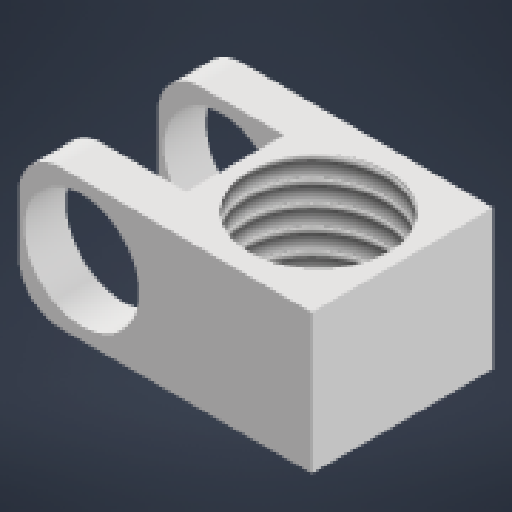
# Autodesk Inventor part: konik
Saved by Autodesk Inventor 2027 (Build 310192060, 192F)
## iProperties
Created: 2026-05-26
Part Number: konik
Material: Ogólny
Document SubType Name: Modeling
Designer: User
Density: 1 g/cm^3
Appearance: Domyślna
Author: User
Autodesk Inventor part; units mm, degrees
ref_plane "YZ Plane" through (0, 0, 0) normal (1, 0, 0) x (0, 1, 0)
ref_plane "XZ Plane" through (0, 0, 0) normal (0, 1, 0) x (-1, 0, 0)
ref_plane "XY Plane" through (0, 0, 0) normal (0, 0, 1) x (1, 0, 0)
sketch "Szkic1" plane through (0, 0, 0) normal (0, 1, 0) x (-1, 0, 0)
  circle A0 centre (0, 0) radius 5
  line L0 (-6, 6.5) -> (6, 6.5)
  line L1 (6, 6.5) -> (6, -6.5)
  line L2 (6, -6.5) -> (-6, -6.5)
  line L3 (-6, -6.5) -> (-6, 6.5)
  line L4 (-6, 6.5) -> (6, -6.5) construction
  line L5 (6, 6.5) -> (-6, -6.5) construction
  line L6 (6, 6.5) -> (15, 6.5)
  line L7 (15, 6.5) -> (15, 3.5)
  line L8 (15, 3.5) -> (6, 3.5)
  line L9 (6, 3.5) -> (6, 6.5)
  line L10 (6, -6.5) -> (15, -6.5)
  line L11 (15, -6.5) -> (15, -3.5)
  line L12 (15, -3.5) -> (6, -3.5)
  line L13 (6, -3.5) -> (6, -6.5)
  dimension "d0" = 10
  dimension "d1" = 12
  dimension "d2" = 13
  dimension "d8" = 9
  dimension "d9" = 3
  dimension "d10" = 3
  constraints: 28 end point, 6 parallel, 3 horizontal, 3 perpendicular, 2 midpoint, 1 centre point, 1 coincident, 1 point on line
  measures "d0" diameter of A0
  measures "d1" distance of L1.end L2.end
  measures "d2" distance of L0.end L1.end
  measures "d8" distance of L7.end L8.end
  measures "d9" distance of L6.end L7.end
  measures "d10" distance of L11.end L10.end
extrude "Wyciągnięcie proste1" add sketch "Szkic1" along normal blind 10
thread "Gwint1" size "M10x1.5" class "6H" standard "ANSI Metric M Profile" full length
sketch "Szkic2" plane through (-15, 0, 6.5) normal (0, 0, 1) x (1, 0, 0)
  line L0 (0, 0) -> (0, 10) projected
  line L1 (0, 5) -> (9, 5)
  line L2 (9, 0) -> (9, 10) projected
  circle A0 centre (4.5, 5) radius 4.1
  point P0 (15, 0)
  dimension "d11" = 8.2
  constraints: 3 midpoint, 2 end point, 1 centre point
  measures "d11" diameter of A0
extrude "Wyciągnięcie proste2" cut sketch "Szkic2" against normal blind 16.75
fillet "Zaokrąglenie2" radius 3 4 edges at (-15, 10, -5) (-15, 0, -5) (-15, 0, 5) (-15, 10, 5)
